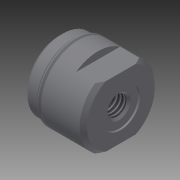
# Autodesk Inventor part: D-14216rear_head
Saved by Autodesk Inventor 2014 (Build 180170000, 170)
## iProperties
Created: 2014-01-19
Part Number: D-14216rear_head
Material: Generic
Catalog Web Link: www.cadenas.de
Description: Rear Head Cyl-Original Line Cyl
Vendor: BIMBA
Document SubType Name: Standard Catalog Part
Designer: Michael
Manufacturer: BIMBA
Density: 1 g/cm^3
Appearance: RGB(211.00000262260440,211.00000262260440,211.00000262260440)
Category: PARTsolutions
Company: BIMBA
Title: D-14216rear_head
Author: Cadenas PARTsolutions
Comments: Original Line Cyl
PSOL_IDENT_0: {$CADENAS_DATA\23d-libs\bimba\bimba\bimba_imperial\bimba_full_line\original_line_cylinders\three_pos
PSOL_IDENT_1: ition_cylinders\rear_head_cyl.prj},184 {VTYP=3D},{NB=D-14216rear_head},{LINA=D-14216rear_head},{NN=R
PSOL_IDENT_2: ear Head Cyl},{DATE=20.08.2011 07:16:50},{GEOMDATE=02.08.2011 10:58:00},{VERSION=},{LINEID=10},{LINE
PSOL_IDENT_3: SUBID=-1},{WBVAR=Q,K}  {NB=D-14216rear_head},{LINA=D-14216rear_head},{KT=DUMMY},{PN=D-14216},{Q=},{Q
PSOL_IDENT_4: ALG='','N/A'},{K=},{KALG= '', 'Standard' , 'K' , 'Ports Rotated 90deg' },{TYPE=1},{ADDER=0.00000000}
PSOL_IDENT_5: ,{A=0.50000000},{AA=0.00000000},{A1=0.18800000},{A11=0.00000000},{A2=0.29700000},{A3=0.01500000},{A4=
PSOL_IDENT_6: 0.18500000},{A5=0.02500000},{A6=0.13200000},{A7=0.18500000},{A8=0.11200000},{B=0.61000000},{BB=0.495
PSOL_IDENT_7: 00000},{B1=0.52300000},{B2=0.57300000},{B3=0.37500000},{B4=0.31200000},{D=0.19000000},{DD=0.00000000
PSOL_IDENT_8: },{CH=0.03000000},{CH1=0.02500000},{CH2=0.01000000},{A111=1.15600000},{A55=0.02500000},{C=0.00000000
PSOL_IDENT_9: },{C1=0.00000000},{C11=0.00000000},{C2=0.00000000},{C21=0.00000000},{C22=0.00000000},{C3=0.00000000}
PSOL_IDENT_10: ,{CCH=0.00000000},{CD=0.00000000},{CDD=0.00000000},{RP=0.02185660},{NDM=0.43750},{CD1=0.43550},{CDD1=
PSOL_IDENT_11: 0.06000},{G=0.10000},{G1=0.03900},{G2=0.03150},{BD=0.00000000}
CNS_NN: Rear Head Cyl
CNS_NT: Original Line Cyl
CNS_NB: D-14216rear_head
CNS_NBSYN: $PN.$Q.$K.rear_head
CNS_LINA: D-14216rear_head
CNS_PN: D-14216
CNS_Q: N/A
CNS_QALG: '','N/A'
CNS_K: Standard
CNS_KALG: '', 'Standard' , 'K' , 'Ports Rotated 90deg'
CNS_TYPE: 1
CNS_ADDER: 0.00000000
CNS_A: 0.50000000
CNS_AA: 0.00000000
CNS_A1: 0.18800000
CNS_A11: 0.00000000
CNS_A2: 0.29700000
CNS_A3: 0.01500000
CNS_A4: 0.18500000
CNS_A5: 0.02500000
CNS_A6: 0.13200000
CNS_A7: 0.18500000
CNS_A8: 0.11200000
CNS_B: 0.61000000
CNS_BB: 0.49500000
CNS_B1: 0.52300000
CNS_B2: 0.57300000
CNS_B3: 0.37500000
CNS_B4: 0.31200000
CNS_D: 0.19000000
CNS_DD: 0.00000000
CNS_CH: 0.03000000
CNS_CH1: 0.02500000
CNS_CH2: 0.01000000
CNS_A111: 1.15600000
CNS_A55: 0.02500000
CNS_C: 0.00000000
CNS_C1: 0.00000000
CNS_C11: 0.00000000
CNS_C2: 0.00000000
CNS_C21: 0.00000000
CNS_C22: 0.00000000
CNS_C3: 0.00000000
CNS_CCH: 0.00000000
CNS_CD: 0.00000000
CNS_CDD: 0.00000000
CNS_RP: 0.02185660
CNS_NDM: 0.43750
CNS_CD1: 0.43550
CNS_CDD1: 0.06000
CNS_G: 0.10000
CNS_G1: 0.03900
CNS_G2: 0.03150
CNS_BD: 0.00000000
SUPPLIER: BIMBA
ARTICLENO: D-14216rear_head
BOMINFO: D-14216rear_head
CREATOR: CADENAS GmbH
Autodesk Inventor part; units mm, degrees
ref_plane "YZ Plane" through (0, 0, 0) normal (1, 0, 0) x (0, 1, 0)
ref_plane "XZ Plane" through (0, 0, 0) normal (0, 1, 0) x (-1, 0, 0)
ref_plane "XY Plane" through (0, 0, 0) normal (0, 0, 1) x (1, 0, 0)
sketch "Sketch_1" plane through (0, 0, 0) normal (0, 0, 1) x (1, 0, 0)
  line L0 (12.7, 0) -> (0, 0)
  line L1 (0, 0) -> (0, 6.5151)
  line L2 (0, 6.5151) -> (0.762, 7.2771)
  line L3 (0.762, 7.2771) -> (2.7178, 7.2771)
  line L4 (2.7178, 7.2771) -> (3.3528, 6.6421)
  line L5 (3.3528, 6.6421) -> (3.9878, 6.6421)
  line L6 (3.9878, 6.6421) -> (3.9878, 7.747)
  line L7 (3.9878, 7.747) -> (11.938, 7.747)
  line L8 (11.938, 7.747) -> (12.7, 6.985)
  line L9 (12.7, 6.985) -> (12.7, 0)
  line L10 (12.7, 0) -> (0, 0)
  constraints: 22 end point
revolve "Revolution1" add sketch "Sketch_1" angle 360 about axis through (12.7, 0, 0) along (1, 0, 0)
sketch "Sketch_2" plane through (12.7, 0, 0) normal (1, 0, 0) x (0, 0, -1)
  line L0 (-30.988, 12.573) -> (-30.988, -12.573)
  line L1 (-30.988, -12.573) -> (30.988, -12.573)
  line L2 (30.988, -12.573) -> (30.988, 12.573)
  line L3 (30.988, 12.573) -> (-30.988, 12.573)
  line L4 (-15.494, 6.2865) -> (-15.494, -6.2865)
  line L5 (-15.494, -6.2865) -> (15.494, -6.2865)
  line L6 (15.494, -6.2865) -> (15.494, 6.2865)
  line L7 (15.494, 6.2865) -> (-15.494, 6.2865)
  constraints: 16 end point
extrude "Extrusion1" cut sketch "Sketch_2" against normal blind 4.699
sketch "Sketch3" plane through (0, 0, 0) normal (-1, 0, 0) x (0, 0, 1)
  point P0 (0, 0)
hole "Hole1" at (0, 0, 0) direction (1, 0, 0) diameter 9.525 depth 4.7752 countersink diameter 10.033 countersink angle 90
sketch "Sketch_5" plane through (0, 0, 0) normal (0, 0, 1) x (1, 0, 0)
  line L0 (12.7, 0) -> (-0.381, 0)
  line L1 (-0.381, 0) -> (-0.381, 1.9837)
  line L2 (-0.381, 1.9837) -> (11.8897, 1.9837)
  line L3 (11.8897, 1.9837) -> (12.319, 2.413)
  line L4 (12.319, 2.413) -> (12.319, 3.9624)
  line L5 (12.319, 3.9624) -> (12.7, 3.9624)
  line L6 (12.7, 3.9624) -> (12.7, 0)
  line L7 (12.7, 0) -> (-0.381, 0)
  constraints: 16 end point
revolve "Revolution2" cut sketch "Sketch_5" angle 360 about axis through (12.7, 0, 0) along (1, 0, 0)
thread "Thread1" size "10-32 UNF" class "2B" standard "ANSI Unified Screw Threads" length 4.699 offset 2.8448
sketch "Sketch_9" plane through (0, 0, 0) normal (0, 0, 1) x (1, 0, 0)
  line L0 (12.7, 0) -> (-12.7, 0)
  line L1 (3.2301, 7.6628) -> (4.2508, 6.6421)
  line L2 (4.2508, 6.6421) -> (4.5382, 6.6421)
  line L3 (4.5382, 6.6421) -> (3.4333, 7.747)
  line L4 (3.4333, 7.747) -> (3.2301, 7.747)
  line L5 (3.2301, 7.747) -> (3.2301, 7.6628)
  constraints: 12 end point
revolve "Revolution3" add sketch "Sketch_9" angle 360 about axis through (12.7, 0, 0) along (1, 0, 0)
ref_plane "aa2_XY" through (12.7, 0, 0) normal (0, 1, 0) x (1, 0, 0)
ref_plane "aa2_YZ" through (12.7, 0, 0) normal (1, 0, 0) x (0, 0, -1)
ref_plane "aa2_ZX" through (12.7, 0, 0) normal (0, 0, -1) x (0, 1, 0)
ref_plane "m1_XY" through (12.7, 0, 0) normal (0, 1, 0) x (1, 0, 0)
ref_plane "m1_YZ" through (12.7, 0, 0) normal (1, 0, 0) x (0, 0, -1)
ref_plane "m1_ZX" through (12.7, 0, 0) normal (0, 0, -1) x (0, 1, 0)
ref_plane "m2_XY" through (8.001, 0, 0) normal (0, 1, 0) x (1, 0, 0)
ref_plane "m2_YZ" through (8.001, 0, 0) normal (1, 0, 0) x (0, 0, -1)
ref_plane "m2_ZX" through (8.001, 0, 0) normal (0, 0, -1) x (0, 1, 0)
ref_plane "n1_XY" through (12.7, 6.2865, 0) normal (1, 0, 0) x (0, 0, -1)
ref_plane "n1_YZ" through (12.7, 6.2865, 0) normal (0, 0, -1) x (0, 1, 0)
ref_plane "n1_ZX" through (12.7, 6.2865, 0) normal (0, 1, 0) x (1, 0, 0)
ref_plane "n2_XY" through (12.7, -6.2865, 0) normal (1, 0, 0) x (0, 0, -1)
ref_plane "n2_YZ" through (12.7, -6.2865, 0) normal (0, 0, -1) x (0, 1, 0)
ref_plane "n2_ZX" through (12.7, -6.2865, 0) normal (0, 1, 0) x (1, 0, 0)
ref_plane "rear_head_XY" through (2.7178, 0, 0) normal (1, 0, 0) x (0, 0, -1)
ref_plane "rear_head_YZ" through (2.7178, 0, 0) normal (0, 0, -1) x (0, 1, 0)
ref_plane "rear_head_ZX" through (2.7178, 0, 0) normal (0, 1, 0) x (1, 0, 0)
ref_plane "to_bushing_XY" through (0, 0, 0) normal (0, 0, 1) x (1, 0, 0)
ref_plane "to_bushing_YZ" through (0, 0, 0) normal (1, 0, 0) x (0, 1, 0)
ref_plane "to_bushing_ZX" through (0, 0, 0) normal (0, 1, 0) x (0, 0, 1)
ref_plane "to_mounting_bracket_xp_XY" through (12.7, 0, 0) normal (1, 0, 0) x (0, 0, -1)
ref_plane "to_mounting_bracket_xp_YZ" through (12.7, 0, 0) normal (0, 0, -1) x (0, 1, 0)
ref_plane "to_mounting_bracket_xp_ZX" through (12.7, 0, 0) normal (0, 1, 0) x (1, 0, 0)
ref_plane "to_pivot_bracket_XY" through (0, 0, 0) normal (0, 0, 1) x (1, 0, 0)
ref_plane "to_pivot_bracket_YZ" through (0, 0, 0) normal (1, 0, 0) x (0, 1, 0)
ref_plane "to_pivot_bracket_ZX" through (0, 0, 0) normal (0, 1, 0) x (0, 0, 1)
body "Solid1"
